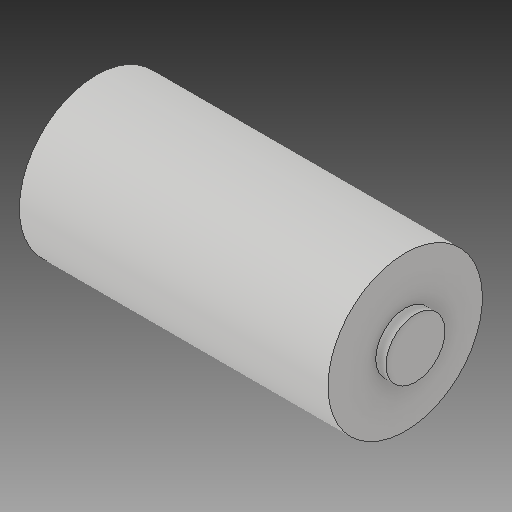
# Autodesk Inventor part: CR123A
Saved by Autodesk Inventor 2017 (Build 210142000, 142)
## iProperties
Part Number: CR123A
Material: 一般
Document SubType Name: Modeling
Designer: sktom
Density: 1 g/cm^3
Appearance: 既定
Author: sktom
Autodesk Inventor part; units mm, degrees
ref_plane "YZ Plane" through (0, 0, 0) normal (1, 0, 0) x (0, 1, 0)
ref_plane "XZ Plane" through (0, 0, 0) normal (0, 1, 0) x (-1, 0, 0)
ref_plane "XY Plane" through (0, 0, 0) normal (0, 0, 1) x (1, 0, 0)
sketch "スケッチ1" plane through (0, 0, 0) normal (0, 0, 1) x (1, 0, 0)
  line L0 (0.5, 0) -> (0.5, 5.95)
  line L1 (0.5, 5.95) -> (0, 5.95)
  line L2 (0, 5.95) -> (0, 8.25)
  line L3 (0, 8.25) -> (33, 8.25)
  line L4 (33, 8.25) -> (33, 3.15)
  line L5 (33, 3.15) -> (34.1, 3.15)
  line L6 (34.1, 3.15) -> (34.1, 0)
  line L7 (34.1, 0) -> (0.5, 0)
  point P0 (0, 0)
  dimension "d0" = 5.95
  dimension "d1" = 8.25
  dimension "d2" = 0.5
  dimension "d3" = 33
  dimension "d4" = 34.1
  dimension "d5" = 3.15
  constraints: 16 end point, 7 perpendicular, 1 horizontal alignment, 1 vertical, 1 vertical alignment
  measures "d0" distance of L0.start L0.end
  measures "d1" distance between parallel lines of L7 L3
  measures "d2" distance of L0.end L1.end
  measures "d3" distance of L2.end L3.end
  measures "d4" distance between parallel lines of L2 L6
  measures "d5" distance of L5.end L6.end
revolve "回転1" add sketch "スケッチ1" angle 360 about axis through (34.1, 0, 0) along (-1, 0, 0)
